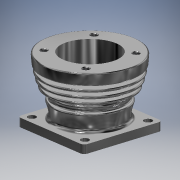
# Autodesk Inventor part: Component 49(Cylinder)
Saved by Autodesk Inventor 2018 (Build 220112000, 112)
## iProperties
Created: 2023-04-10
Part Number: Component 49(Cylinder)
Material: Generic
Document SubType Name: Modeling
Designer: Habib Mohamed
Density: 1 g/cm^3
Appearance: Chrome - Polished Black
Author: Habib Mohamed
Autodesk Inventor part; units mm, degrees
note: some values were not read from the file. Chosen so that the rebuilt part matches the saved one: direction of "Hole1".
ref_plane "YZ Plane" through (0, 0, 0) normal (1, 0, 0) x (0, 1, 0)
ref_plane "XZ Plane" through (0, 0, 0) normal (0, 1, 0) x (-1, 0, 0)
ref_plane "XY Plane" through (0, 0, 0) normal (0, 0, 1) x (1, 0, 0)
sketch "Sketch1" plane through (0, 0, 0) normal (0, 1, 0) x (-1, 0, 0)
  line L0 (18, 20) -> (-18, 20)
  line L1 (-20, 18) -> (-20, -18)
  line L2 (-18, -20) -> (18, -20)
  line L3 (20, -18) -> (20, 18)
  line L4 (20, 20) -> (-20, -20) construction
  line L5 (-20, 20) -> (20, -20) construction
  circle A0 centre (16, 16) radius 2
  circle A1 centre (16, -16) radius 2
  circle A2 centre (-16, 16) radius 2
  circle A3 centre (-16, -16) radius 2
  arc A4 (20, 18) -> (18, 20) centre (18, 18) ccw
  arc A5 (-18, 20) -> (-20, 18) centre (-18, 18) ccw
  arc A6 (-20, -18) -> (-18, -20) centre (-18, -18) ccw
  arc A7 (18, -20) -> (20, -18) centre (18, -18) ccw
  circle A8 centre (0, 0) radius 13.5
  dimension "d0" = 40
  dimension "d1" = 40
  dimension "d2" = 4
  dimension "d3" = 4
  dimension "d4" = 4
  dimension "d5" = 2
  dimension "d6" = 27
  constraints: 12 end point, 12 point on line, 9 centre point, 8 point on circle, 8 tangent, 6 equal radius, 2 midpoint, 2 parallel, 2 vertical alignment, 1 coincident, 1 horizontal, 1 horizontal alignment, 1 perpendicular
  measures "d0" distance of L5.end L4.start
  measures "d1" distance of L4.end L5.end
  measures "d2" diameter of A0
  measures "d3" distance from line of L0 A0.centre
  measures "d4" distance from line of L3 A0.centre
  measures "d5" radius of A4
  measures "d6" diameter of A8
extrude "Extrusion1" add sketch "Sketch1" along normal blind 4
sketch "Sketch2" plane through (0, 0, 0) normal (0, 0, 1) x (1, 0, 0)
  line L0 (-20, 0) -> (-20, 4) construction
  line L1 (-20, 4) -> (-13.5, 4) construction
  line L2 (-13.5, 4) -> (-13.5, 0) construction
  line L3 (-13.5, 0) -> (-20, 0) projected
  line L4 (20, 4) -> (20, 0) projected
  line L5 (20, 0) -> (13.5, 0) projected
  line L6 (13.5, 0) -> (13.5, 4) projected
  line L7 (13.5, 4) -> (20, 4) projected
  line L8 (-13.5, 4) -> (13.5, 4) construction
  line L9 (0, 4) -> (0, 32) construction
  arc A0 (-22.9923, 31.2349) -> (-22.6561, 26.8993) centre (15, 32) ccw construction
  line L10 (-13.5, 32) -> (-22.2424, 32) construction
  line L11 (-13.5, 32) -> (-13.5, 4) construction
  circle A1 centre (-16.75, 25.5) radius 0.75 construction
  arc A2 (-16.75, 21.76) -> (-16.75, 23.26) centre (-16.75, 22.51) ccw construction
  arc A3 (-16.75, 18.68) -> (-16.75, 20.18) centre (-16.75, 19.43) ccw construction
  arc A4 (-16.2558, 15.5359) -> (-16, 16.1) centre (-16.75, 16.1) ccw
  arc A5 (-16.2558, 15.5359) -> (-16.2558, 14.4041) centre (-15.76, 14.97) ccw
  arc A6 (-16.7136, 12.7609) -> (-16, 13.51) centre (-16.75, 13.51) ccw
  line L12 (-16.75, 26.25) -> (-21.9129, 26.25) construction
  line L13 (-16.75, 24.75) -> (-21.387, 24.75) construction
  line L14 (-16.75, 23.26) -> (-21.9812, 23.26) construction
  line L15 (-16.75, 21.76) -> (-21.5943, 21.76) construction
  line L16 (-16.75, 20.18) -> (-21.1149, 20.18) construction
  line L17 (-16.75, 18.68) -> (-20.589, 18.68) construction
  line L18 (-16.75, 17.18) -> (-19.991, 17.18) construction
  arc A7 (-16.7136, 12.7609) -> (-17.3729, 11.7315) centre (-16.6772, 12.0118) ccw
  line L19 (-16, 16.43) -> (-16, 16.1)
  line L20 (-16, 13.84) -> (-16, 13.51)
  arc A8 (-16, 16.43) -> (-16.75, 17.18) centre (-16.75, 16.43) ccw
  arc A9 (-16, 13.84) -> (-16.2558, 14.4041) centre (-16.75, 13.84) ccw
  arc A10 (-22.6561, 26.8993) -> (-21.9129, 26.25) centre (-21.9129, 27) ccw construction
  arc A11 (-21.387, 24.75) -> (-21.387, 23.26) centre (-21.387, 24.005) ccw construction
  arc A12 (-20.5376, 21.76) -> (-20.5376, 20.18) centre (-20.5376, 20.97) ccw
  arc A13 (-19.4905, 18.68) -> (-19.4905, 17.18) centre (-19.4905, 17.93) ccw construction
  line L21 (-18, 4) -> (18, 4) construction
  line L22 (-16.0112, 4) -> (-13.5, 4) construction
  arc A14 (-22.2424, 32) -> (-22.9923, 31.2349) centre (-22.2424, 31.25) ccw construction
  arc A15 (-22.6561, 26.8993) -> (-22.1147, 23.8451) centre (15, 32) ccw construction
  arc A16 (-22.1147, 23.8451) -> (-18.2107, 13.5326) centre (15, 32) ccw construction
  line L23 (-16.75, 26.25) -> (-22.5624, 26.25) construction
  line L24 (-13.5, 32) -> (-22.2424, 32)
  arc A17 (-22.2424, 32) -> (-22.2424, 32) centre (-22.2424, 31.2502) ccw
  arc A18 (-22.2424, 32) -> (-22.9923, 31.2349) centre (-22.2424, 31.25) ccw
  arc A19 (-22.9923, 31.2349) -> (-22.6561, 26.8993) centre (15, 32) ccw
  arc A20 (-22.6561, 26.8993) -> (-21.9129, 26.25) centre (-21.9129, 27) ccw
  line L25 (-21.9129, 26.25) -> (-16.75, 26.25)
  line L26 (-16.75, 24.75) -> (-21.387, 24.75)
  line L27 (-21.387, 23.26) -> (-16.75, 23.26)
  line L28 (-16.75, 21.76) -> (-20.5376, 21.76)
  line L29 (-20.5376, 20.18) -> (-16.75, 20.18)
  line L30 (-16.75, 18.68) -> (-19.4905, 18.68)
  line L31 (-19.4905, 17.18) -> (-16.75, 17.18)
  line L32 (-16.0112, 4) -> (-13.5, 4)
  line L33 (-18, 4) -> (-14, 4) projected
  line L34 (-13.5, 4) -> (-13.5, 32)
  arc A21 (-16.75, 24.75) -> (-16.75, 26.25) centre (-16.75, 25.5) ccw
  arc A22 (-16.75, 21.76) -> (-16.75, 23.26) centre (-16.75, 22.51) ccw
  arc A23 (-16.75, 18.68) -> (-16.75, 20.18) centre (-16.75, 19.43) ccw
  arc A24 (-21.387, 24.75) -> (-21.387, 23.26) centre (-21.387, 24.005) ccw
  arc A25 (-19.4905, 18.68) -> (-19.4905, 17.18) centre (-19.4905, 17.93) ccw
  arc A26 (-16.0112, 4) -> (-17.3729, 11.7315) centre (-34.95, 4.65) ccw
  point P0 (0, 0)
  point P1 (-23, 32)
  point P2 (-12.7534, 6.0433)
  point P3 (-16.75, 13.84)
  point P4 (-16.75, 16.1)
  dimension "d29" = 1.5
  dimension "d9" = 32
  dimension "d10" = 4.65
  dimension "d11" = 32
  dimension "d12" = 15
  dimension "d13" = 76
  dimension "d15" = 34.95
  dimension "d16" = 5.75
  dimension "d18" = 0.75
  dimension "d19" = 3.74
  dimension "d20" = 6.82
  dimension "d21" = 9.82
  dimension "d22" = 11.28
  dimension "d23" = 12.41
  dimension "d24" = 12.74
  dimension "d25" = 10.15
  dimension "d26" = 13.5
  dimension "d27" = 3.25
  dimension "d28" = 2.26
  dimension "d30" = 1.5
  dimension "d31" = 1.5
  dimension "d33" = 1.5
  dimension "d36" = 1.5
  dimension "d38" = 1.5
  dimension "d39" = 1.5
  dimension "d40" = 0.75
  constraints: 72 point on circle, 48 end point, 27 tangent, 26 centre point, 11 collinear, 11 horizontal, 11 point on line, 10 coincident, 8 vertical alignment, 5 concentric, 3 vertical, 1 equal radius, 1 midpoint, 2 other
  measures "d9" distance of point (0, 0) L9.end
  measures "d10" vertical distance of point (0, 0) point (-34.95, 4.65)
  measures "d11" vertical distance of point (0, 0) point (15, 32)
  measures "d12" distance of L9.end point (15, 32)
  measures "d13" diameter of A0
  measures "d15" horizontal distance of A26.centre point (0, 0)
  measures "d16" distance from line of L12.start L10
  measures "d18" distance of point (-16.75, 25.5) L12.start
  measures "d19" distance of point (-16.75, 22.51) L12.start
  measures "d20" distance of point (-16.75, 19.43) L12.start
  measures "d21" distance of point (-16.75, 16.43) L12.start
  measures "d22" vertical distance of point (-15.76, 14.97) L12.start
  measures "d23" distance of point (-16.75, 13.84) L12.start
  measures "d24" distance of L12.start point (-16.75, 13.51)
  measures "d25" distance of L12.start point (-16.75, 16.1)
  measures "d26" distance between parallel lines of L9 L11
  measures "d27" distance from line of L11 L12.start
  measures "d28" distance from line of L11 point (-15.76, 14.97)
  measures "d30" diameter of A2
  measures "d31" diameter of A3
  measures "d33" diameter of A4
  measures "d36" diameter of A6
  measures "d38" diameter of A7
  measures "d39" diameter of A10
  measures "d40" radius of A14
revolve "Revolution1" add sketch "Sketch2" angle 360 about axis through (0, 4, 0) along (0, 1, 0) contours A4 L19 A8 L31 A25 L30 A23 L29 A12 L28 A22 L27 A24 L26 A21 L25 A20 A19 A17 L24 L34 L32 A26 A7 A6 L20 A9 A5 | A17
sketch "Sketch3" plane through (0, 32, 0) normal (0, 1, 0) x (1, 0, 0)
  line L0 (0, 0) -> (-41.413, 41.413) construction
  circle A0 centre (0, 0) radius 18 construction
  line L1 (0, 0) -> (0, 50.2716) construction
  point P0 (-12.7279, 12.7279)
  point P1 (-12.7279, -12.7279)
  point P2 (12.7279, -12.7279)
  point P3 (12.7279, 12.7279)
  dimension "d42" = 36
  dimension "d43" = 45
  dimension "d46" = 360
  constraints: 4 end point, 1 coincident, 1 point on line, 1 vertical, 8 other
  measures "d43" angle of L0 L1
hole "Hole1" at (-12.7279, 32, -12.7279) at (-12.7279, 32, 12.7279) at (12.7279, 32, 12.7279) at (12.7279, 32, -12.7279) direction (0, -1, 0) diameter 3.242 end up to surface thread size "M4x0.7" class "6H" standard "ISO Metric profile"
chamfer "Chamfer1" distance 0.3 angle 45 4 edges at (-12.7279, 32, -14.3489) (-12.7279, 32, 11.1069) (12.7279, 32, 11.1069) (12.7279, 32, -14.3489)
fillet "Fillet1" radius 2 1 edges at (16.0112, 4, 0)
body "Solid1"
